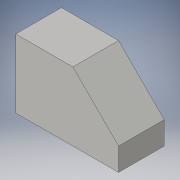
# Autodesk Inventor part: Figure 7_27_9
Saved by Autodesk Inventor 2016 (Build 200138000, 138)
## iProperties
Created: 2016-07-19
Part Number: Figure 7_27_9
Material: Generic
Document SubType Name: Modeling
Designer: cfkguest
Density: 1 g/cm^3
Appearance: Default
Author: cfkguest
Autodesk Inventor part; units mm, degrees
ref_plane "YZ Plane" through (0, 0, 0) normal (1, 0, 0) x (0, 1, 0)
ref_plane "XZ Plane" through (0, 0, 0) normal (0, 1, 0) x (-1, 0, 0)
ref_plane "XY Plane" through (0, 0, 0) normal (0, 0, 1) x (1, 0, 0)
sketch "Sketch1" plane through (0, 0, 0) normal (0, 0, 1) x (1, 0, 0)
  line L0 (-10.0399, 22.4932) -> (47.1101, 22.4932)
  line L1 (47.1101, 22.4932) -> (47.1101, -15.6068)
  line L2 (47.1101, -15.6068) -> (-10.0399, -15.6068)
  line L3 (-10.0399, -15.6068) -> (-10.0399, 22.4932)
  point P0 (0, 0)
  dimension "d0" = 57.15
  dimension "d1" = 38.1
  constraints: 8 end point, 2 parallel, 1 horizontal, 1 perpendicular
  measures "d0" distance of L0.start L0.end
  measures "d1" distance of L2.end L0.start
extrude "Extrusion1" add sketch "Sketch1" along normal blind 25.4
chamfer "Chamfer1" distance 25.4 angle 45 1 edges at (47.1101, 22.4932, 12.7)
body "Solid1"
